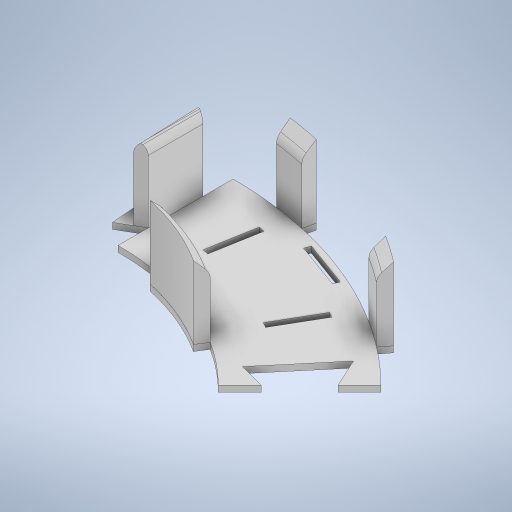
# Autodesk Inventor part: Moving Carousel Upper
Saved by Autodesk Inventor 2023 (Build 270158000, 158)
## iProperties
Created: 2023-02-15
Part Number: Moving Carousel Upper
Material: Generic
Document SubType Name: Modeling
Designer: cheng
Density: 1 g/cm^3
Appearance: Default
Author: cheng
Autodesk Inventor part; units mm, degrees
ref_plane "YZ Plane" through (0, 0, 0) normal (1, 0, 0) x (0, 1, 0)
ref_plane "XZ Plane" through (0, 0, 0) normal (0, 1, 0) x (-1, 0, 0)
ref_plane "XY Plane" through (0, 0, 0) normal (0, 0, 1) x (1, 0, 0)
sketch "Sketch1" plane through (0, 0, 0) normal (0, 1, 0) x (-1, 0, 0)
  circle A0 centre (0, 0) radius 215
  circle A1 centre (0, 0) radius 280
  circle A2 centre (0, 0) radius 200
  circle A3 centre (0, 0) radius 295
  circle A4 centre (0, 0) radius 270
  circle A5 centre (0, 0) radius 225
  line L0 (0, 0) -> (0, -295)
  line L1 (0, 0) -> (-208.5965, -208.5965)
  line L2 (0, 0) -> (-189.6223, -225.9831)
  line L3 (0, 0) -> (25.7109, -293.8774)
  line L4 (24.4036, -278.9345) -> (0, -270)
  line L5 (18.7385, -214.1819) -> (0, -225)
  line L6 (-138.1993, -164.6996) -> (-159.099, -159.099)
  line L7 (-179.9805, -214.4924) -> (-190.9188, -190.9188)
  line L8 (0, 0) -> (-100.8959, -277.2093) construction
  circle A6 centre (0, 0) radius 235 construction
  circle A7 centre (0, 0) radius 275 construction
  circle A8 centre (0, 0) radius 325 construction
  circle A9 centre (0, 0) radius 255 construction
  circle A10 centre (0, 0) radius 285 construction
  line L9 (-80.392, -279.3513) -> (-117.9797, -265.6705)
  line L10 (-117.9797, -265.6705) -> (-116.2696, -260.972)
  line L11 (-116.2696, -260.972) -> (-78.6819, -274.6528)
  line L12 (-78.6819, -274.6528) -> (-80.392, -279.3513)
  line L13 (-80.392, -279.3513) -> (-116.2696, -260.972) construction
  line L14 (-117.9797, -265.6705) -> (-78.6819, -274.6528) construction
  line L15 (-98.3308, -270.1616) -> (-99.1858, -272.5109) construction
  line L16 (-139.6651, -236.907) -> (-135.335, -239.407)
  line L17 (-135.335, -239.407) -> (-115.335, -204.766)
  line L18 (-115.335, -204.766) -> (-119.6651, -202.266)
  line L19 (-119.6651, -202.266) -> (-139.6651, -236.907)
  line L20 (-139.6651, -236.907) -> (-115.335, -204.766) construction
  line L21 (-135.335, -239.407) -> (-119.6651, -202.266) construction
  line L22 (-137.5, -238.157) -> (-117.5, -203.516) construction
  circle A11 centre (0, 0) radius 275 construction
  line L23 (-45.2912, -271.2563) -> (-50.2152, -270.388)
  line L24 (-50.2152, -270.388) -> (-43.2693, -230.9957)
  line L25 (-43.2693, -230.9957) -> (-38.3453, -231.8639)
  line L26 (-38.3453, -231.8639) -> (-45.2912, -271.2563)
  line L27 (-45.2912, -271.2563) -> (-43.2693, -230.9957) construction
  line L28 (-50.2152, -270.388) -> (-38.3453, -231.8639) construction
  line L29 (-47.7532, -270.8221) -> (-40.8073, -231.4298) construction
  circle A12 centre (0, 0) radius 165 construction
  point P0 (0, -200)
  point P1 (-141.4214, -141.4214)
  point P2 (23.5321, -268.9726)
  point P3 (-127.5, -220.8365)
  point P4 (-44.2803, -251.126)
  dimension "d3" = 430
  dimension "d5" = 15
  dimension "d7" = 45
  dimension "d8" = 5
  dimension "d9" = 5
  dimension "d10" = 10
  dimension "d12" = 10
  dimension "d15" = 20
  dimension "d18" = 590
  dimension "d19" = 650
  dimension "d20" = 90
  dimension "d24" = 20
  dimension "d29" = 5
  dimension "d30" = 40
  dimension "d33" = 5
  dimension "d34" = 40
  dimension "d37" = 40
  dimension "d41" = 330
  dimension "d42" = 35
  dimension "d45" = 10
  constraints: 60 end point, 13 point on circle, 12 centre point, 12 coincident, 8 point on line, 7 midpoint, 7 symmetric about line, 4 parallel, 3 tangent, 2 perpendicular, 1 collinear, 1 vertical, 4 other
  measures "d3" diameter of A0
  measures "d5" radial gap between concentric circles of A1 A3
  measures "d7" angle of L0 L1
  measures "d8" angle of L1 L2
  measures "d9" angle of L3 L0
  measures "d10" radial gap between concentric circles of A0 A5
  measures "d12" radial gap between concentric circles of A1 A4
  measures "d15" angle of L2 L8
  measures "d18" diameter of A3
  measures "d19" diameter of A8
  measures "d20" radial gap between concentric circles of A8 A6
  measures "d29" distance between parallel lines of L9 L11
  measures "d30" distance between parallel lines of L10 L12
  measures "d33" distance between parallel lines of L19 L17
  measures "d34" distance between parallel lines of L16 L18
  measures "d37" radial gap between concentric circles of A8 A10
  measures "d41" diameter of A12
  measures "d42" radial gap between concentric circles of A2 A12
  measures "d45" angle of L17 L8
extrude "Extrusion1" add sketch "Sketch1" along normal blind 5 contours L3 A5 L5 | L0 A5 L2 A0 | A0 L2 A2 L0 | L3 A4 L0 A5 | L0 A4 L26 L25 L24 L17 L18 L19 L2 A5 | L1 A2 L2 A0 | A0 L6 L1 | L3 L4 A4 | L0 A1 L2 A4 L19 L16 L17 L24 L23 L26 | L0 A3 L2 A1 | L7 A1 L1 | L2 A3 L1 A1
sketch "Sketch2" plane through (0, 0, 0) normal (0, -1, 0) x (1, 0, 0)
  line L0 (179.9805, -214.4924) -> (190.9188, -190.9188) projected
  line L1 (190.9188, -190.9188) -> (208.5965, -208.5965) projected
  arc A0 (0, -295) -> (208.5965, -208.5965) centre (0, 0) ccw projected
  line L2 (0, -295) -> (0, -270) projected
  line L3 (0, -270) -> (-24.4036, -278.9345) projected
  line L4 (-24.4036, -278.9345) -> (-18.7385, -214.1819) projected
  line L5 (-18.7385, -214.1819) -> (0, -225) projected
  line L6 (0, -225) -> (0, -200) projected
  arc A1 (0, -200) -> (141.4214, -141.4214) centre (0, 0) ccw projected
  line L7 (141.4214, -141.4214) -> (159.099, -159.099) projected
  line L8 (159.099, -159.099) -> (138.1993, -164.6996) projected
  line L9 (138.1993, -164.6996) -> (179.9805, -214.4924) projected
  line L10 (115.335, -204.766) -> (135.335, -239.407) projected
  line L11 (135.335, -239.407) -> (139.6651, -236.907) projected
  line L12 (139.6651, -236.907) -> (119.6651, -202.266) projected
  line L13 (119.6651, -202.266) -> (115.335, -204.766) projected
  line L14 (50.2152, -270.388) -> (43.2693, -230.9957) projected
  line L15 (43.2693, -230.9957) -> (38.3453, -231.8639) projected
  line L16 (38.3453, -231.8639) -> (45.2912, -271.2563) projected
  line L17 (45.2912, -271.2563) -> (50.2152, -270.388) projected
  line L18 (80.392, -279.3513) -> (117.9797, -265.6705) projected
  line L19 (117.9797, -265.6705) -> (116.2696, -260.972) projected
  line L20 (116.2696, -260.972) -> (78.6819, -274.6528) projected
  line L21 (78.6819, -274.6528) -> (80.392, -279.3513) projected
  circle A2 centre (0, 0) radius 200
  circle A3 centre (0, 0) radius 295
  circle A4 centre (0, 0) radius 305
  circle A5 centre (0, 0) radius 190
  line L22 (0, 0) -> (51.7638, -193.1852)
  arc A6 (0, -200) -> (141.4214, -141.4214) centre (0, 0) ccw projected
  line L23 (0, 0) -> (100, -173.2051)
  line L24 (0, 0) -> (39.8105, -302.3907)
  line L25 (0, 0) -> (66.0141, -297.7703)
  line L26 (0, 0) -> (163.8764, -257.2344)
  line L27 (0, 0) -> (185.6722, -241.9728)
  line L28 (0, 0) -> (116.7184, -281.7833) construction
  line L29 (0, 0) -> (0, -305) construction
  point P0 (41.1235, -185.4962)
  point P1 (43.2879, -195.2592)
  point P2 (107.4599, -168.6783)
  point P3 (102.0869, -160.2444)
  point P4 (179.5846, -234.0392)
  point P5 (158.5034, -248.8005)
  point P6 (63.8497, -288.0073)
  point P7 (38.5052, -292.4762)
  dimension "d46" = 10
  dimension "d47" = 10
  dimension "d50" = 15
  dimension "d51" = 5
  dimension "d52" = 5
  dimension "d53" = 22.5
  dimension "d54" = 10
  dimension "d55" = 10
  dimension "d56" = 7.5
  constraints: 16 end point, 8 point on circle, 4 centre point, 4 coincident, 2 concentric, 1 vertical
  measures "d46" radial gap between concentric circles of A5 A2
  measures "d47" radial gap between concentric circles of A0 A4
  measures "d50" angle of L23 L22
  measures "d51" angle of L25 L24
  measures "d52" angle of L27 L26
  measures "d53" angle of L29 L28
  measures "d54" angle of L25 L28
  measures "d55" angle of L28 L26
  measures "d56" angle of L28 L22
extrude "Extrusion2" add sketch "Sketch2" against normal blind 5 contours L27 A4 L26 A0 | L25 A4 L24 A0 | A1 L23 A5 L26 | L25 A5 L22 A1 | A1 L22 A5 L23
sketch "Sketch3" plane through (0, 5, 0) normal (0, 1, 0) x (1, 0, 0)
  line L0 (179.9805, 214.4924) -> (190.9188, 190.9188) projected
  line L1 (190.9188, 190.9188) -> (208.5965, 208.5965) projected
  arc A0 (208.5965, 208.5965) -> (179.5846, 234.0392) centre (0, 0) ccw projected
  line L2 (179.5846, 234.0392) -> (185.6722, 241.9728) projected
  arc A1 (185.6722, 241.9728) -> (163.8764, 257.2344) centre (0, 0) ccw projected
  line L3 (163.8764, 257.2344) -> (158.5034, 248.8005) projected
  arc A2 (158.5034, 248.8005) -> (63.8497, 288.0073) centre (0, 0) ccw projected
  line L4 (63.8497, 288.0073) -> (66.0141, 297.7703) projected
  arc A3 (66.0141, 297.7703) -> (39.8105, 302.3907) centre (0, 0) ccw projected
  line L5 (39.8105, 302.3907) -> (38.5052, 292.4762) projected
  arc A4 (38.5052, 292.4762) -> (0, 295) centre (0, 0) ccw projected
  line L6 (0, 295) -> (0, 270) projected
  line L7 (0, 270) -> (-24.4036, 278.9345) projected
  line L8 (-24.4036, 278.9345) -> (-18.7385, 214.1819) projected
  line L9 (-18.7385, 214.1819) -> (0, 225) projected
  line L10 (0, 225) -> (0, 200) projected
  arc A5 (43.2879, 195.2592) -> (0, 200) centre (0, 0) ccw projected
  line L11 (43.2879, 195.2592) -> (41.1235, 185.4962) projected
  arc A6 (102.0869, 160.2444) -> (41.1235, 185.4962) centre (0, 0) ccw projected
  line L12 (102.0869, 160.2444) -> (107.4599, 168.6783) projected
  arc A7 (141.4214, 141.4214) -> (107.4599, 168.6783) centre (0, 0) ccw projected
  line L13 (141.4214, 141.4214) -> (159.099, 159.099) projected
  line L14 (159.099, 159.099) -> (138.1993, 164.6996) projected
  line L15 (138.1993, 164.6996) -> (179.9805, 214.4924) projected
  line L16 (115.335, 204.766) -> (135.335, 239.407) projected
  line L17 (135.335, 239.407) -> (139.6651, 236.907) projected
  line L18 (139.6651, 236.907) -> (119.6651, 202.266) projected
  line L19 (119.6651, 202.266) -> (115.335, 204.766) projected
  line L20 (50.2152, 270.388) -> (43.2693, 230.9957) projected
  line L21 (43.2693, 230.9957) -> (38.3453, 231.8639) projected
  line L22 (38.3453, 231.8639) -> (45.2912, 271.2563) projected
  line L23 (45.2912, 271.2563) -> (50.2152, 270.388) projected
  line L24 (80.392, 279.3513) -> (117.9797, 265.6705) projected
  line L25 (117.9797, 265.6705) -> (116.2696, 260.972) projected
  line L26 (116.2696, 260.972) -> (78.6819, 274.6528) projected
  line L27 (78.6819, 274.6528) -> (80.392, 279.3513) projected
  circle A8 centre (0, 0) radius 190
  circle A9 centre (0, 0) radius 200
  circle A10 centre (0, 0) radius 295
  circle A11 centre (0, 0) radius 305
  line L28 (0, 0) -> (43.2879, 195.2592)
  line L29 (0, 0) -> (107.4599, 168.6783)
  line L30 (0, 0) -> (39.8105, 302.3907)
  line L31 (0, 0) -> (66.0141, 297.7703)
  line L32 (0, 0) -> (163.8764, 257.2344)
  line L33 (0, 0) -> (185.6722, 241.9728)
  line L34 (0, 0) -> (0, 305)
  line L35 (0, 0) -> (-10.6443, 304.8142)
  point P0 (43.2879, 195.2592)
  point P1 (179.5846, 234.0392)
  point P2 (63.8497, 288.0073)
  point P3 (-9.5507, 273.4967)
  point P4 (-7.7019, 220.5535)
  dimension "d59" = 2
  constraints: 16 end point, 4 coincident, 3 centre point, 3 concentric, 2 collinear, 2 point on circle, 1 vertical, 3 other
  measures "d59" angle of L35 L34
extrude "Extrusion3" add sketch "Sketch3" along normal blind 60 separate body contours A10 L3 A1 L2 | A10 L5 A3 L4 | L12 A6 L11 A9 | L7 L34 L9 L35
chamfer "Chamfer1" distance 10 angle 45 3 edges at (51.2262, 65, -290.5183) (76.5367, 65, -184.7759) (169.205, 65, -241.6499)
fillet "Fillet1" radius 10 3 edges at (51.2262, 55.0005, -290.5183) (169.205, 55.0005, -241.6499) (76.5367, 55.0005, -184.7759)
chamfer "Chamfer2" distance 4 angle 45 2 edges at (0, 65, -247.5) (-8.6263, 65, -247.0251)
fillet "Fillet2" radius 10 2 edges at (0, 61, -247.5) (-8.6263, 61, -247.0251)
body "Solid1"
body "Solid2"
